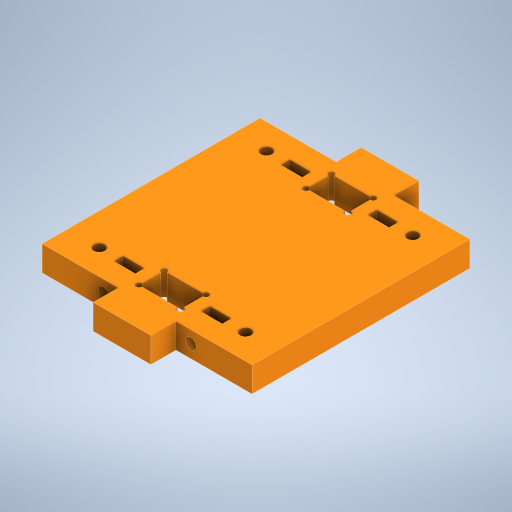
# Autodesk Inventor part: bridge1
Saved by Autodesk Inventor 2024 (Build 280153000, 153)
## iProperties
Created: 2024-09-05
Part Number: bridge1
Material: PMMA 플라스틱
Document SubType Name: Modeling
Designer: jmha0
Density: 1.188 g/cm^3
Appearance: 주황색
Mass: 14.4768 g
Surface Area: 66.3237 cm^2
Volume: 12.1859 cm^3
Author: jmha0
Autodesk Inventor part; units mm, degrees
ref_plane "YZ Plane" through (0, 0, 0) normal (1, 0, 0) x (0, 1, 0)
ref_plane "XZ Plane" through (0, 0, 0) normal (0, 1, 0) x (-1, 0, 0)
ref_plane "XY Plane" through (0, 0, 0) normal (0, 0, 1) x (1, 0, 0)
sketch "스케치1" plane through (0, 0, 0) normal (0, 1, 0) x (-1, 0, 0)
  line L0 (0, 0) -> (27.8, 0)
  line L1 (27.8, 0) -> (27.8, -52.1)
  line L2 (27.8, -52.1) -> (0, -52.1)
  line L3 (0, -52.1) -> (0, 0)
  line L4 (27.8, 0) -> (20.8, 0)
  line L5 (20.8, 0) -> (7, 0)
  line L6 (20.8, 0) -> (7, 0)
  line L7 (7, 0) -> (7, 6)
  line L8 (7, 6) -> (20.8, 6)
  line L9 (20.8, 6) -> (20.8, 0)
  line L10 (20.8, -52.1) -> (7, -52.1)
  line L11 (7, -52.1) -> (7, -58.1)
  line L12 (7, -58.1) -> (20.8, -58.1)
  line L13 (20.8, -58.1) -> (20.8, -52.1)
  line L14 (-20.5978, 0) -> (-48.3978, 0)
  line L15 (-48.3978, -52.1) -> (-20.5978, -52.1)
  line L16 (-34.4978, -52.1) -> (-27.5978, -52.1)
  line L17 (-27.5978, -52.1) -> (-41.3978, -52.1)
  line L18 (-41.3978, -52.1) -> (-41.3978, -58.1)
  line L19 (-41.3978, -58.1) -> (-27.5978, -58.1)
  line L20 (-27.5978, -58.1) -> (-27.5978, -52.1)
  line L21 (-27.5978, 0) -> (-41.3978, 0)
  line L22 (-41.3978, 0) -> (-41.3978, 6)
  line L23 (-41.3978, 6) -> (-27.5978, 6)
  line L24 (-27.5978, 6) -> (-27.5978, 0)
  line L25 (-20.5978, -52.1) -> (-14.5978, -52.1)
  line L26 (-14.5978, -52.1) -> (-14.5978, 0)
  line L27 (-14.5978, 0) -> (-20.5978, 0)
  line L28 (-48.3978, -52.1) -> (-54.3978, -52.1)
  line L29 (-54.3978, -52.1) -> (-54.3978, 0)
  line L30 (-54.3978, 0) -> (-48.3978, 0)
  line L31 (-48.3978, 0) -> (-48.3978, -52.1)
  point P0 (-27.5978, 3)
  point P1 (-41.3978, 3)
  dimension "d0" = 27.8
  dimension "d1" = 52.1
  dimension "d2" = 7
  dimension "d4" = 13.8
  dimension "d5" = 6
  dimension "d6" = 6
  dimension "d33" = 27.8
  dimension "d34" = 52.1
  dimension "d35" = 6.9
  dimension "d36" = 13.8
  dimension "d37" = 13.8
  dimension "d59" = 6
  dimension "d60" = 6
  constraints: 64 end point, 14 parallel, 9 point on line, 8 horizontal, 7 perpendicular, 3 midpoint
  measures "d0" distance of L1.end L2.end
  measures "d1" distance of L0.end L1.end
  measures "d2" distance of L0.end L4.end
  measures "d4" distance of L4.end L5.end
  measures "d5" distance of L6.end L7.end
  measures "d6" distance of L11.end L10.end
  measures "d33" distance of L15.end L15.start
  measures "d34" distance of L15.start L14.end
  measures "d35" distance of L16.start L16.end
  measures "d36" distance of L19.end L18.end
  measures "d37" distance of L22.end L23.end
  measures "d59" distance of L27.end L26.end
  measures "d60" distance of L29.end L30.end
extrude "돌출1" add sketch "스케치1" along normal blind 6 contours L27 L26 L25 L15 L31 L14 | L14 L22 L23 L24 | L31 L28 L29 L30 | L20 L19 L18 L15
sketch "스케치25" plane through (14.5978, 0, 0) normal (0, 0, 1) x (1, 0, 0)
  circle A0 centre (9.5, 3) radius 1.35 projected
  circle A1 centre (30.3, 3) radius 1.35 projected
  point P0 (-14.5978, 0)
extrude "돌출21" cut sketch "스케치25" against normal blind 10
sketch "스케치26" plane through (54.3978, 0, -52.1) normal (0, 0, -1) x (-1, 0, 0)
  circle A0 centre (9.5, 3) radius 1.35 projected
  circle A1 centre (30.3, 3) radius 1.35 projected
  point P0 (54.3978, 0)
extrude "돌출22" cut sketch "스케치26" against normal blind 10
sketch "스케치27" plane through (0, 6, 0) normal (0, 1, 0) x (1, 0, 0)
  line L0 (27.5978, 52.1) -> (14.5978, 52.1) projected
  line L1 (27.5978, 52.1) -> (14.5978, 52.1) projected
  line L2 (27.5978, 58.1) -> (27.5978, 52.1) projected
  line L3 (27.5978, 52.1) -> (14.5978, 52.1) projected
  line L4 (14.5978, 52.1) -> (14.5978, 0) projected
  line L5 (14.5978, 0) -> (27.5978, 0) projected
  line L6 (27.5978, 0) -> (27.5978, -6) projected
  line L7 (27.5978, -6) -> (41.3978, -6) projected
  line L8 (41.3978, -6) -> (41.3978, 0) projected
  line L9 (41.3978, 0) -> (54.3978, 0) projected
  line L10 (54.3978, 0) -> (54.3978, 52.1) projected
  line L11 (54.3978, 52.1) -> (41.3978, 52.1) projected
  line L12 (41.3978, 52.1) -> (41.3978, 58.1) projected
  line L13 (41.3978, 58.1) -> (27.5978, 58.1) projected
  line L14 (27.5978, 58.1) -> (27.5978, 52.1) projected
  line L15 (41.3978, 58.1) -> (27.5978, 58.1) projected
  line L16 (41.3978, 52.1) -> (41.3978, 58.1) projected
  line L17 (54.3978, 52.1) -> (41.3978, 52.1) projected
  line L18 (54.3978, 0) -> (54.3978, 52.1) projected
  line L19 (41.3978, 0) -> (54.3978, 0) projected
  line L20 (41.3978, -6) -> (41.3978, 0) projected
  line L21 (27.5978, -6) -> (41.3978, -6) projected
  line L22 (27.5978, 0) -> (27.5978, -6) projected
  line L23 (14.5978, 0) -> (27.5978, 0) projected
  line L24 (14.5978, 52.1) -> (14.5978, 0) projected
  line L25 (27.5978, 52.1) -> (14.5978, 52.1) projected
  line L26 (14.5978, 52.1) -> (14.5978, 0) projected
  line L27 (14.5978, 52.1) -> (14.5978, 0) projected
  line L28 (14.5978, 52.1) -> (14.5978, 0) projected
  line L29 (14.5978, 52.1) -> (14.5978, 0) projected
  line L30 (54.3978, 0) -> (54.3978, 52.1) projected
  line L31 (54.3978, 0) -> (54.3978, 52.1) projected
  line L32 (54.3978, 0) -> (54.3978, 52.1) projected
  line L33 (54.3978, 0) -> (54.3978, 52.1) projected
  line L34 (22.7478, 42.1) -> (25.4478, 42.1) projected
  line L35 (22.7478, 42.1) -> (25.4478, 42.1) projected
  line L36 (43.5478, 42.1) -> (46.2478, 42.1) projected
  line L37 (43.5478, 52.1) -> (46.2478, 52.1) projected
  line L38 (43.5478, 52.1) -> (46.2478, 52.1) projected
  line L39 (54.3978, 52.1) -> (41.3978, 52.1) projected
  line L40 (54.3978, 52.1) -> (41.3978, 52.1) projected
  line L41 (43.5478, 52.1) -> (46.2478, 52.1) projected
  line L42 (54.3978, 52.1) -> (41.3978, 52.1) projected
  line L43 (54.3978, 52.1) -> (41.3978, 52.1) projected
  line L44 (43.5478, 42.1) -> (46.2478, 42.1) projected
  line L45 (43.5478, 42.1) -> (46.2478, 42.1) projected
  line L46 (22.7478, 52.1) -> (25.4478, 52.1) projected
  line L47 (22.7478, 52.1) -> (25.4478, 52.1) projected
  line L48 (27.5978, 52.1) -> (14.5978, 52.1) projected
  line L49 (27.5978, 52.1) -> (14.5978, 52.1) projected
  line L50 (46.2478, 10) -> (43.5478, 10) projected
  line L51 (46.2478, 10) -> (43.5478, 10) projected
  line L52 (46.2478, 10) -> (43.5478, 10) projected
  line L53 (46.2478, 0) -> (43.5478, 0) projected
  line L54 (25.4478, 10) -> (22.7478, 10) projected
  line L55 (25.4478, 10) -> (22.7478, 10) projected
  line L56 (41.3978, -6) -> (41.3978, 0) projected
  line L57 (41.3978, -6) -> (41.3978, 0) projected
  line L58 (41.3978, -6) -> (41.3978, 0) projected
  line L59 (41.3978, -6) -> (41.3978, 0) projected
  line L60 (25.4478, 10) -> (22.7478, 10) projected
  line L61 (25.4478, 0) -> (22.7478, 0) projected
  line L62 (25.4478, 0) -> (22.7478, 0) projected
  line L63 (27.5978, 0) -> (27.5978, -6) projected
  line L64 (27.5978, 0) -> (27.5978, -6) projected
  line L65 (27.5978, 0) -> (27.5978, -6) projected
  line L66 (14.5978, 0) -> (27.5978, 0) projected
  line L67 (14.5978, 0) -> (27.5978, 0) projected
  line L68 (25.4478, 0) -> (22.7478, 0) projected
  line L69 (14.5978, 0) -> (27.5978, 0) projected
  line L70 (14.5978, 0) -> (27.5978, 0) projected
  line L71 (27.5978, 0) -> (27.5978, -6) projected
  line L72 (46.2478, 0) -> (43.5478, 0) projected
  line L73 (41.3978, 0) -> (54.3978, 0) projected
  line L74 (41.3978, 0) -> (54.3978, 0) projected
  line L75 (46.2478, 0) -> (43.5478, 0) projected
  line L76 (41.3978, 0) -> (54.3978, 0) projected
  line L77 (41.3978, 0) -> (54.3978, 0) projected
  line L78 (22.7478, 42.1) -> (25.4478, 42.1) projected
  line L79 (22.7478, 52.1) -> (25.4478, 52.1) projected
  line L80 (27.5978, -6) -> (41.3978, -6) projected
  line L81 (27.5978, -6) -> (41.3978, -6) projected
  line L82 (27.5978, -6) -> (41.3978, -6) projected
  line L83 (27.5978, -6) -> (41.3978, -6) projected
  line L84 (27.5978, 58.1) -> (27.5978, 52.1) projected
  line L85 (27.5978, 58.1) -> (27.5978, 52.1) projected
  line L86 (27.5978, 58.1) -> (27.5978, 52.1) projected
  line L87 (27.5978, 58.1) -> (27.5978, 52.1) projected
  line L88 (41.3978, 58.1) -> (27.5978, 58.1) projected
  line L89 (41.3978, 58.1) -> (27.5978, 58.1) projected
  line L90 (41.3978, 58.1) -> (27.5978, 58.1) projected
  line L91 (41.3978, 58.1) -> (27.5978, 58.1) projected
  line L92 (41.3978, 52.1) -> (41.3978, 58.1) projected
  line L93 (41.3978, 52.1) -> (41.3978, 58.1) projected
  line L94 (41.3978, 52.1) -> (41.3978, 58.1) projected
  line L95 (41.3978, 52.1) -> (41.3978, 58.1) projected
  line L96 (22.7478, 52.1) -> (22.7478, 42.1) projected
  line L97 (25.4478, 52.1) -> (25.4478, 42.1) projected
  line L98 (43.5478, 52.1) -> (43.5478, 42.1) projected
  line L99 (46.2478, 52.1) -> (46.2478, 42.1) projected
  line L100 (46.2478, 0) -> (46.2478, 10) projected
  line L101 (43.5478, 0) -> (43.5478, 10) projected
  line L102 (25.4478, 0) -> (25.4478, 10) projected
  line L103 (22.7478, 0) -> (22.7478, 10) projected
  line L104 (44.8978, 0) -> (44.8978, 6.1)
  line L105 (47.4978, 5) -> (42.2978, 5)
  line L106 (42.2978, 5) -> (42.2978, 7.2)
  line L107 (42.2978, 7.2) -> (47.4978, 7.2)
  line L108 (47.4978, 7.2) -> (47.4978, 5)
  line L109 (47.4978, 5) -> (42.2978, 7.2) construction
  line L110 (42.2978, 5) -> (47.4978, 7.2) construction
  line L111 (26.6978, 5) -> (21.4978, 5)
  line L112 (21.4978, 5) -> (21.4978, 7.2)
  line L113 (21.4978, 7.2) -> (26.6978, 7.2)
  line L114 (26.6978, 7.2) -> (26.6978, 5)
  line L115 (26.6978, 5) -> (21.4978, 7.2) construction
  line L116 (21.4978, 5) -> (26.6978, 7.2) construction
  line L117 (44.8978, 52.1) -> (44.8978, 46)
  line L118 (47.4978, 47.1) -> (42.2978, 47.1)
  line L119 (42.2978, 47.1) -> (42.2978, 44.9)
  line L120 (42.2978, 44.9) -> (47.4978, 44.9)
  line L121 (47.4978, 44.9) -> (47.4978, 47.1)
  line L122 (47.4978, 47.1) -> (42.2978, 44.9) construction
  line L123 (42.2978, 47.1) -> (47.4978, 44.9) construction
  line L124 (26.6978, 47.1) -> (21.4978, 47.1)
  line L125 (21.4978, 47.1) -> (21.4978, 44.9)
  line L126 (21.4978, 44.9) -> (26.6978, 44.9)
  line L127 (26.6978, 44.9) -> (26.6978, 47.1)
  line L128 (26.6978, 47.1) -> (21.4978, 44.9) construction
  line L129 (21.4978, 47.1) -> (26.6978, 44.9) construction
  point P0 (0, 0)
  point P1 (24.0978, 6.1)
  point P2 (24.0978, 46)
  dimension "d183" = 6.1
  dimension "d184" = 5.2
  dimension "d185" = 2.2
  dimension "d186" = 5.2
  dimension "d187" = 2.2
  dimension "d188" = 6.1
  dimension "d189" = 5.2
  dimension "d190" = 2.2
  dimension "d191" = 5.2
  dimension "d192" = 2.2
  constraints: 52 end point, 9 parallel, 8 midpoint, 5 perpendicular, 4 horizontal, 2 point on line, 6 other
  measures "d183" distance of L104.start L104.end
  measures "d184" distance of L106.end L107.end
  measures "d185" distance of L105.end L106.end
  measures "d186" distance of L112.end L113.end
  measures "d187" distance of L111.end L112.end
  measures "d188" distance of L117.start L117.end
  measures "d189" distance of L120.end L119.end
  measures "d190" distance of L119.end L118.end
  measures "d191" distance of L126.end L125.end
  measures "d192" distance of L125.end L124.end
extrude "돌출23" cut sketch "스케치27" against normal blind 10 contours L124 L127 L126 L97 | L97 L126 L96 L124 | L96 L126 L125 L124 | L118 L99 L120 L98 | L98 L120 L119 L118 | L111 L112 L113 L103 | L103 L113 L102 L111 | L102 L113 L114 L111 | L118 L121 L120 L99 | L105 L101 L107 L100 | L100 L107 L108 L105 | L105 L106 L107 L101
sketch "스케치28" plane through (0, 6, 0) normal (0, 1, 0) x (1, 0, 0)
  line L0 (26.6978, 47.1) -> (26.6978, 44.9) projected
  line L1 (26.6978, 44.9) -> (21.4978, 44.9) projected
  line L2 (21.4978, 44.9) -> (21.4978, 47.1) projected
  line L3 (21.4978, 47.1) -> (26.6978, 47.1) projected
  line L4 (21.4978, 5) -> (21.4978, 7.2) projected
  line L5 (21.4978, 7.2) -> (26.6978, 7.2) projected
  line L6 (26.6978, 7.2) -> (26.6978, 5) projected
  line L7 (26.6978, 5) -> (21.4978, 5) projected
  line L8 (47.4978, 47.1) -> (47.4978, 44.9) projected
  line L9 (47.4978, 44.9) -> (42.2978, 44.9) projected
  line L10 (42.2978, 44.9) -> (42.2978, 47.1) projected
  line L11 (42.2978, 47.1) -> (47.4978, 47.1) projected
  line L12 (42.2978, 5) -> (42.2978, 7.2) projected
  line L13 (42.2978, 7.2) -> (47.4978, 7.2) projected
  line L14 (47.4978, 7.2) -> (47.4978, 5) projected
  line L15 (47.4978, 5) -> (42.2978, 5) projected
  line L16 (27.5978, 58.1) -> (27.5978, 52.1) projected
  line L17 (27.5978, 52.1) -> (14.5978, 52.1) projected
  line L18 (14.5978, 52.1) -> (14.5978, 0) projected
  line L19 (14.5978, 0) -> (27.5978, 0) projected
  line L20 (27.5978, 0) -> (27.5978, -6) projected
  line L21 (27.5978, -6) -> (41.3978, -6) projected
  line L22 (41.3978, -6) -> (41.3978, 0) projected
  line L23 (41.3978, 0) -> (54.3978, 0) projected
  line L24 (54.3978, 0) -> (54.3978, 52.1) projected
  line L25 (54.3978, 52.1) -> (41.3978, 52.1) projected
  line L26 (41.3978, 52.1) -> (41.3978, 58.1) projected
  line L27 (41.3978, 58.1) -> (27.5978, 58.1) projected
  line L28 (14.5978, 0) -> (27.5978, 0) projected
  line L29 (14.5978, 0) -> (14.3978, 0)
  line L30 (14.3978, 0) -> (14.3978, 52.1)
  line L31 (14.3978, 52.1) -> (14.5978, 52.1)
  line L32 (14.5978, 52.1) -> (14.5978, 0)
  line L33 (54.3978, 0) -> (54.5978, 0)
  line L34 (54.5978, 0) -> (54.5978, 52.1)
  line L35 (54.5978, 52.1) -> (54.3978, 52.1)
  line L36 (54.3978, 52.1) -> (54.3978, 0)
  point P0 (0, 0)
  dimension "d195" = 39.8
  dimension "d196" = 0.2
  dimension "d197" = 0.2
  constraints: 16 end point, 4 parallel, 2 horizontal, 2 perpendicular, 1 point on line
  measures "d195" distance between parallel lines of L18 L24
  measures "d196" distance of L30.end L31.end
  measures "d197" distance of L35.end L34.end
extrude "돌출24" add sketch "스케치28" against normal blind 6 contours L18 L29 L30 L31 | L35 L34 L33 L24
sketch "스케치29" plane through (0, 6, 0) normal (0, 1, 0) x (1, 0, 0)
  line L0 (39.4978, 49.05) -> (39.4978, 43.05)
  line L1 (39.4978, 43.05) -> (54.5978, 43.05)
  line L2 (54.5978, 43.05) -> (54.5978, 49.05)
  line L3 (39.4978, 49.05) -> (54.5978, 49.05)
  line L4 (29.4978, 49.05) -> (39.4978, 49.05)
  line L5 (29.4978, 49.05) -> (29.4978, 43.05)
  line L6 (39.4978, 43.05) -> (29.4978, 43.05)
  line L7 (39.4978, 49.05) -> (39.4978, 43.05)
  line L8 (39.4978, 9.05) -> (39.4978, 3.05)
  line L9 (54.5978, 3.05) -> (39.4978, 3.05)
  line L10 (54.5978, 9.05) -> (54.5978, 3.05)
  line L11 (54.5978, 9.05) -> (39.4978, 9.05)
  line L12 (39.4978, 3.05) -> (29.4978, 3.05)
  line L13 (39.4978, 3.05) -> (39.4978, 9.05)
  line L14 (29.4978, 9.05) -> (39.4978, 9.05)
  line L15 (29.4978, 3.05) -> (29.4978, 9.05)
  line L16 (29.4978, 3.05) -> (29.4978, 9.05)
  line L17 (29.4978, 9.05) -> (14.3978, 9.05)
  line L18 (14.3978, 9.05) -> (14.3978, 3.05)
  line L19 (29.4978, 3.05) -> (14.3978, 3.05)
  line L20 (29.4978, 43.05) -> (29.4978, 49.05)
  line L21 (14.3978, 49.05) -> (29.4978, 49.05)
  line L22 (14.3978, 43.05) -> (14.3978, 49.05)
  line L23 (14.3978, 43.05) -> (29.4978, 43.05)
  line L24 (26.6978, 47.1) -> (26.6978, 44.9) projected
  line L25 (26.6978, 44.9) -> (21.4978, 44.9) projected
  line L26 (21.4978, 44.9) -> (21.4978, 47.1) projected
  line L27 (21.4978, 47.1) -> (26.6978, 47.1) projected
  line L28 (21.4978, 5) -> (21.4978, 7.2) projected
  line L29 (21.4978, 7.2) -> (26.6978, 7.2) projected
  line L30 (26.6978, 7.2) -> (26.6978, 5) projected
  line L31 (26.6978, 5) -> (21.4978, 5) projected
  line L32 (47.4978, 47.1) -> (47.4978, 44.9) projected
  line L33 (47.4978, 44.9) -> (42.2978, 44.9) projected
  line L34 (42.2978, 44.9) -> (42.2978, 47.1) projected
  line L35 (42.2978, 47.1) -> (47.4978, 47.1) projected
  line L36 (42.2978, 5) -> (42.2978, 7.2) projected
  line L37 (42.2978, 7.2) -> (47.4978, 7.2) projected
  line L38 (47.4978, 7.2) -> (47.4978, 5) projected
  line L39 (47.4978, 5) -> (42.2978, 5) projected
  line L40 (27.5978, 58.1) -> (27.5978, 52.1) projected
  line L41 (27.5978, 52.1) -> (14.3978, 52.1) projected
  line L42 (14.3978, 52.1) -> (14.3978, 0) projected
  line L43 (14.3978, 0) -> (27.5978, 0) projected
  line L44 (27.5978, 0) -> (27.5978, -6) projected
  line L45 (27.5978, -6) -> (41.3978, -6) projected
  line L46 (41.3978, -6) -> (41.3978, 0) projected
  line L47 (41.3978, 0) -> (54.5978, 0) projected
  line L48 (54.5978, 0) -> (54.5978, 52.1) projected
  line L49 (54.5978, 52.1) -> (41.3978, 52.1) projected
  line L50 (41.3978, 52.1) -> (41.3978, 58.1) projected
  line L51 (41.3978, 58.1) -> (27.5978, 58.1) projected
  line L52 (54.5978, 9.05) -> (14.3978, 9.05)
  line L53 (14.3978, 9.05) -> (14.3978, 43.05)
  line L54 (14.3978, 43.05) -> (54.5978, 43.05)
  line L55 (54.5978, 43.05) -> (54.5978, 9.05)
  point P0 (0, 0)
  constraints: 56 end point, 2 parallel, 1 horizontal, 1 perpendicular
extrude "돌출25" cut sketch "스케치29" against normal blind 6 contours L0 L6 L5 L4 | L8 L12 L15 L14
sketch "스케치30" plane through (0, 6, 0) normal (0, 1, 0) x (1, 0, 0)
  line L0 (46.2478, 10) -> (43.5478, 10) projected
  line L1 (39.4978, 43.05) -> (29.4978, 43.05) projected
  line L2 (29.4978, 43.05) -> (29.4978, 49.05) projected
  line L3 (29.4978, 49.05) -> (39.4978, 49.05) projected
  line L4 (39.4978, 49.05) -> (39.4978, 43.05) projected
  line L5 (29.4978, 9.05) -> (39.4978, 9.05) projected
  line L6 (39.4978, 9.05) -> (39.4978, 3.05) projected
  line L7 (39.4978, 3.05) -> (29.4978, 3.05) projected
  line L8 (29.4978, 3.05) -> (29.4978, 9.05) projected
  line L9 (26.6978, 47.1) -> (26.6978, 44.9) projected
  line L10 (26.6978, 44.9) -> (21.4978, 44.9) projected
  line L11 (21.4978, 44.9) -> (21.4978, 47.1) projected
  line L12 (21.4978, 47.1) -> (26.6978, 47.1) projected
  line L13 (21.4978, 5) -> (21.4978, 7.2) projected
  line L14 (21.4978, 7.2) -> (26.6978, 7.2) projected
  line L15 (26.6978, 7.2) -> (26.6978, 5) projected
  line L16 (26.6978, 5) -> (21.4978, 5) projected
  line L17 (47.4978, 47.1) -> (47.4978, 44.9) projected
  line L18 (47.4978, 44.9) -> (42.2978, 44.9) projected
  line L19 (42.2978, 44.9) -> (42.2978, 47.1) projected
  line L20 (42.2978, 47.1) -> (47.4978, 47.1) projected
  line L21 (42.2978, 5) -> (42.2978, 7.2) projected
  line L22 (42.2978, 7.2) -> (47.4978, 7.2) projected
  line L23 (47.4978, 7.2) -> (47.4978, 5) projected
  line L24 (47.4978, 5) -> (42.2978, 5) projected
  line L25 (27.5978, 58.1) -> (27.5978, 52.1) projected
  line L26 (27.5978, 52.1) -> (14.3978, 52.1) projected
  line L27 (14.3978, 52.1) -> (14.3978, 0) projected
  line L28 (14.3978, 0) -> (27.5978, 0) projected
  line L29 (27.5978, 0) -> (27.5978, -6) projected
  line L30 (27.5978, -6) -> (41.3978, -6) projected
  line L31 (41.3978, -6) -> (41.3978, 0) projected
  line L32 (41.3978, 0) -> (54.5978, 0) projected
  line L33 (54.5978, 0) -> (54.5978, 52.1) projected
  line L34 (54.5978, 52.1) -> (41.3978, 52.1) projected
  line L35 (41.3978, 52.1) -> (41.3978, 58.1) projected
  line L36 (41.3978, 58.1) -> (27.5978, 58.1) projected
  line L37 (54.5978, 0) -> (54.5978, 3.05)
  line L38 (54.5978, 52.1) -> (54.5978, 49.05)
  line L39 (54.5978, 3.05) -> (49.3978, 3.05)
  line L40 (49.3978, 3.05) -> (49.3978, 9.05)
  line L41 (49.3978, 9.05) -> (54.5978, 9.05)
  line L42 (54.5978, 9.05) -> (54.5978, 3.05)
  line L43 (14.3978, 0) -> (14.3978, 52.1) projected
  line L44 (14.3978, 8.05) -> (14.3978, 2.05)
  line L45 (54.5978, 49.05) -> (49.3978, 49.05)
  line L46 (49.3978, 49.05) -> (49.3978, 43.05)
  line L47 (49.3978, 43.05) -> (54.5978, 43.05)
  line L48 (54.5978, 43.05) -> (54.5978, 49.05)
  line L49 (14.3978, 49.05) -> (19.5978, 49.05)
  line L50 (19.5978, 49.05) -> (19.5978, 43.05)
  line L51 (19.5978, 43.05) -> (14.3978, 43.05)
  line L52 (14.3978, 43.05) -> (14.3978, 49.05)
  circle A0 centre (51.9978, 46.05) radius 1.35
  circle A1 centre (16.9978, 46.05) radius 1.35
  circle A2 centre (51.9978, 6.05) radius 1.35
  line L53 (14.3978, 3.05) -> (19.5978, 3.05)
  line L54 (19.5978, 3.05) -> (19.5978, 9.05)
  line L55 (19.5978, 9.05) -> (14.3978, 9.05)
  line L56 (14.3978, 9.05) -> (14.3978, 3.05)
  circle A3 centre (16.9978, 6.05) radius 1.35
  point P0 (0, 0)
  dimension "d202" = 3.05
  dimension "d203" = 3.05
  dimension "d204" = 5.2
  dimension "d205" = 6
  dimension "d210" = 5.2
  dimension "d211" = 6
  dimension "d212" = 5.2
  dimension "d213" = 6
  dimension "d218" = 2.7
  dimension "d219" = 2.7
  dimension "d220" = 2.7
  dimension "d222" = 5.2
  dimension "d223" = 6
  dimension "d224" = 2.7
  constraints: 38 end point, 8 parallel, 6 point on line, 4 centre point, 4 horizontal, 4 perpendicular
  measures "d202" distance of L32.end L37.end
  measures "d203" distance of L33.end L38.end
  measures "d204" distance of L40.end L41.end
  measures "d205" distance of L39.end L40.end
  measures "d210" distance of L47.end L46.end
  measures "d211" distance of L46.end L45.end
  measures "d212" distance of L50.end L51.end
  measures "d213" distance of L49.end L50.end
  measures "d218" diameter of A0
  measures "d219" diameter of A1
  measures "d220" diameter of A2
  measures "d222" distance of L55.end L54.end
  measures "d223" distance of L54.end L53.end
  measures "d224" diameter of A3
extrude "돌출26" cut sketch "스케치30" against normal blind 6 contours A0 | A1 | A2 | A3
sketch "스케치31" plane through (0, 6, 0) normal (0, 1, 0) x (1, 0, 0)
  circle A0 centre (51.9978, 46.05) radius 1.35 projected
  circle A1 centre (51.9978, 6.05) radius 1.35 projected
  circle A2 centre (16.9978, 46.05) radius 1.35 projected
  circle A3 centre (16.9978, 6.05) radius 1.35 projected
  line L0 (39.4978, 43.05) -> (29.4978, 43.05) projected
  line L1 (29.4978, 43.05) -> (29.4978, 49.05) projected
  line L2 (29.4978, 49.05) -> (39.4978, 49.05) projected
  line L3 (39.4978, 49.05) -> (39.4978, 43.05) projected
  line L4 (29.4978, 9.05) -> (39.4978, 9.05) projected
  line L5 (39.4978, 9.05) -> (39.4978, 3.05) projected
  line L6 (39.4978, 3.05) -> (29.4978, 3.05) projected
  line L7 (29.4978, 3.05) -> (29.4978, 9.05) projected
  line L8 (26.6978, 47.1) -> (26.6978, 44.9) projected
  line L9 (26.6978, 44.9) -> (21.4978, 44.9) projected
  line L10 (21.4978, 44.9) -> (21.4978, 47.1) projected
  line L11 (21.4978, 47.1) -> (26.6978, 47.1) projected
  line L12 (21.4978, 5) -> (21.4978, 7.2) projected
  line L13 (21.4978, 7.2) -> (26.6978, 7.2) projected
  line L14 (26.6978, 7.2) -> (26.6978, 5) projected
  line L15 (26.6978, 5) -> (21.4978, 5) projected
  line L16 (47.4978, 47.1) -> (47.4978, 44.9) projected
  line L17 (47.4978, 44.9) -> (42.2978, 44.9) projected
  line L18 (42.2978, 44.9) -> (42.2978, 47.1) projected
  line L19 (42.2978, 47.1) -> (47.4978, 47.1) projected
  line L20 (42.2978, 5) -> (42.2978, 7.2) projected
  line L21 (42.2978, 7.2) -> (47.4978, 7.2) projected
  line L22 (47.4978, 7.2) -> (47.4978, 5) projected
  line L23 (47.4978, 5) -> (42.2978, 5) projected
  line L24 (27.5978, 58.1) -> (27.5978, 52.1) projected
  line L25 (27.5978, 52.1) -> (14.3978, 52.1) projected
  line L26 (14.3978, 52.1) -> (14.3978, 0) projected
  line L27 (14.3978, 0) -> (27.5978, 0) projected
  line L28 (27.5978, 0) -> (27.5978, -6) projected
  line L29 (27.5978, -6) -> (41.3978, -6) projected
  line L30 (41.3978, -6) -> (41.3978, 0) projected
  line L31 (41.3978, 0) -> (54.5978, 0) projected
  line L32 (54.5978, 0) -> (54.5978, 52.1) projected
  line L33 (54.5978, 52.1) -> (41.3978, 52.1) projected
  line L34 (41.3978, 52.1) -> (41.3978, 58.1) projected
  line L35 (41.3978, 58.1) -> (27.5978, 58.1) projected
  circle A4 centre (29.4978, 49.05) radius 0.75
  circle A5 centre (39.4978, 49.05) radius 0.75
  circle A6 centre (39.4978, 43.05) radius 0.75
  line L36 (39.4978, 43.05) -> (29.4978, 43.05) projected
  circle A7 centre (29.4978, 43.05) radius 0.75
  circle A8 centre (29.4978, 9.05) radius 0.75
  circle A9 centre (39.4978, 9.05) radius 0.75
  circle A10 centre (39.4978, 3.05) radius 0.75
  circle A11 centre (29.4978, 3.05) radius 0.75
  point P0 (0, 0)
  dimension "d225" = 1.5
  dimension "d226" = 1.5
  dimension "d227" = 1.5
  dimension "d228" = 1.5
  dimension "d229" = 1.5
  dimension "d230" = 1.5
  dimension "d231" = 1.5
  dimension "d232" = 1.5
  constraints: 8 centre point, 8 coincident
  measures "d225" diameter of A4
  measures "d226" diameter of A5
  measures "d227" diameter of A6
  measures "d228" diameter of A7
  measures "d229" diameter of A8
  measures "d230" diameter of A9
  measures "d231" diameter of A10
  measures "d232" diameter of A11
extrude "돌출27" cut sketch "스케치31" against normal blind 6 contours A7 L1 L0 | L0 L1 A7 | A6 L3 L0 | L0 L3 A6 | A4 L2 L1 | L1 L2 A4 | A5 L2 L3 | L3 L2 A5 | L7 A8 L4 | L4 A8 L7 | A9 L5 L4 | L4 L5 A9 | A11 L6 L7 | L7 L6 A11 | A10 L6 L5 | L5 L6 A10
sketch "스케치32" plane through (54.5978, 6, 0) normal (1, 0, 0) x (0, 0, -1)
  line L0 (0, 0) -> (52.1, 0) projected
  line L1 (0, 0) -> (0, -6) projected
  line L2 (52.1, -6) -> (0, -6) projected
  line L3 (52.1, 0) -> (52.1, -6) projected
extrude "돌출28" add sketch "스케치32" along normal blind 5
sketch "스케치33" plane through (14.3978, 6, -52.1) normal (-1, 0, 0) x (0, 0, 1)
  line L0 (0, 0) -> (52.1, 0) projected
  line L1 (0, 0) -> (0, -6) projected
  line L2 (52.1, -6) -> (0, -6) projected
  line L3 (52.1, 0) -> (52.1, -6) projected
extrude "돌출29" add sketch "스케치33" along normal blind 5
